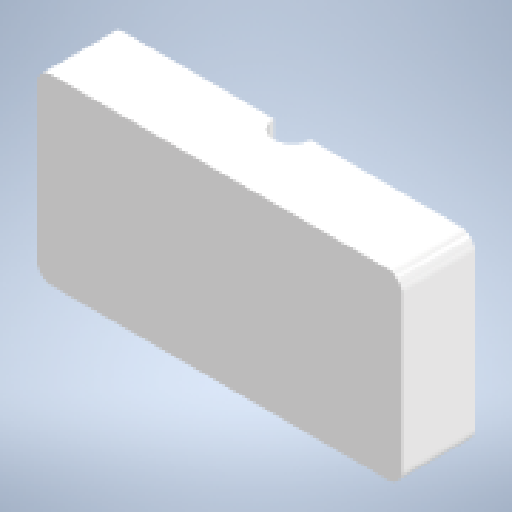
# Autodesk Inventor part: TrittOT
Saved by Autodesk Inventor 2024.4 (Build 284460000, 460)
## iProperties
Created: 2026-01-10
Part Number: TrittOT
Material: PVC, hart
Description: TrittOT
Document SubType Name: Modeling
Designer: Philf
Mass: 115.836 g
Surface Area: 171.616 cm^2
Volume: 89.7954 cm^3
Density: 1.29 g/cm^3
Appearance: Glatt - Weiß
Masse[kg]: 0,100 kg
Author: Philf
Autodesk Inventor part; units mm, degrees
ref_plane "YZ Plane" through (0, 0, 0) normal (1, 0, 0) x (0, 1, 0)
ref_plane "XZ Plane" through (0, 0, 0) normal (0, 1, 0) x (-1, 0, 0)
ref_plane "XY Plane" through (0, 0, 0) normal (0, 0, 1) x (1, 0, 0)
sketch "Skizze1" plane through (0, 0, 0) normal (0, 1, 0) x (-1, 0, 0)
  line L0 (0, 0) -> (0, -50)
  line L1 (0, -50) -> (100, -50)
  line L2 (100, -50) -> (100, 0)
  line L3 (100, 0) -> (0, 0)
  dimension "d0" = 50
  dimension "d1" = 100
  constraints: 8 end point, 3 perpendicular, 1 vertical
  measures "d0" distance of L0.start L0.end
  measures "d1" distance of L0.end L1.end
extrude "Extrusion1" add sketch "Skizze1" along normal blind 20
fillet "Rundung1" radius 4 4 edges at (0, 10, 0) (0, 10, -50) (-100, 10, -50) (-100, 10, 0)
sketch "Skizze2" plane through (-96, 0, 0) normal (0, 0, 1) x (1, 0, 0)
  line L0 (0, 20) -> (0, 0) projected
  line L1 (0, 0) -> (46, 0)
  line L2 (0, 0) -> (92, 0) projected
  line L3 (46, 0) -> (46, 20)
  circle A0 centre (46, 20) radius 10
  point P0 (96, 0)
  dimension "d5" = 46
  dimension "d6" = 20
  dimension "d7" = 20
  constraints: 4 end point, 1 centre point, 1 coincident, 1 midpoint, 1 perpendicular
  measures "d5" distance of L0.end L1.end
  measures "d6" distance of L1.end L3.end
  measures "d7" diameter of A0
extrude "Extrusion2" cut sketch "Skizze2" against normal through all
sketch "Skizze3" plane through (0, 0, 0) normal (0, -1, 0) x (1, 0, 0)
  line L0 (0, 0) -> (0, -10)
  line L1 (0, -4) -> (0, -46) projected
  line L2 (0, -10) -> (-15, -10)
  line L3 (-15, -10) -> (-85, -10)
  line L4 (-85, -10) -> (-85, -40)
  line L5 (-85, -40) -> (-15, -40)
  dimension "d10" = 10
  dimension "d11" = 15
  dimension "d12" = 70
  dimension "d13" = 30
  constraints: 10 end point, 3 perpendicular, 2 point on line
  measures "d10" distance of L0.start L0.end
  measures "d11" distance of L0.end L2.end
  measures "d12" distance of L2.end L3.end
  measures "d13" distance of L3.end L4.end
hole "Bohrung1" at (-85, 0, -40) at (-85, 0, -10) at (-15, 0, -40) at (-15, 0, -10) direction (0, 1, 0) diameter 5.2 end through all countersink diameter 11 countersink angle 90
equation "\"d0\" = breite"
equation "\"d1\" = länge"
equation "\"d4\" = radius"
equation "\"d7\" = durchmesser"
equation "\"breite\" = 50"
equation "\"länge\" = 100"
equation "\"radius\" = 4"
equation "\"durchmesser\" = 20"
